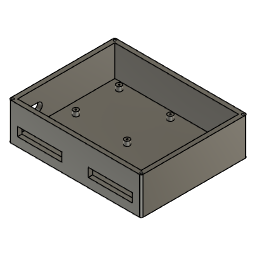
台座 (Autodesk Fusion 360 design; units mm, degrees)
Autodesk Fusion 360 part; units mm, degrees
note: some values were not read from the file. Set by a fixed rule: which sketch regions a step uses.
sketch "スケッチ6" plane through (0, 0, 0) normal (0, 0, 1) x (1, 0, 0)
  line L0 (75, -45) -> (-75, -45)
  line L1 (-75, -45) -> (-75, 75)
  line L2 (-75, 75) -> (75, 75)
  line L3 (75, 75) -> (75, -45)
  line L4 (-200, 0) -> (160, 0)
  dimension "d22" = 150
  dimension "d110" = 75
  dimension "d111" = 45
  constraint horizontal L0
  constraint perpendicular L0 L1
  constraint parallel L0 L2
  constraint parallel L1 L3
  constraint perpendicular L3 L4
  measures "d22" distance of L1.end L2.end
  measures "d110" distance of L2 L4
  measures "d111" distance of L0 L4
extrude "押し出し4" add sketch "スケッチ6" along normal blind 42
sketch "スケッチ7" plane through (0, 0, 42) normal (0, 0, 1) x (-1, 0, 0)
  line L0 (-75, -75) -> (75, -75)
  line L1 (75, -75) -> (75, 45)
  line L2 (75, 45) -> (-75, 45)
  line L3 (-75, 45) -> (-75, -75)
  line L4 (70, -70) -> (-70, -70)
  line L5 (-70, -70) -> (-70, 40)
  line L6 (-70, 40) -> (70, 40)
  line L7 (70, 40) -> (70, -70)
  dimension "d26" = 5
  dimension "d27" = 5
  constraint horizontal L4
  constraint vertical L5
  constraint horizontal L6
  constraint vertical L7
  measures "d26" distance of L2 L6
  measures "d27" distance of L0 L4
extrude "押し出し5" cut sketch "スケッチ7" against normal blind 35 contours L4 L5 L6 L7
sketch "スケッチ8" plane through (0, 0, 7) normal (0, 0, 1) x (-1, 0, 0)
  line L0 (70, 40) -> (-70, 40)
  line L1 (-70, 40) -> (-70, -70)
  line L2 (-70, -70) -> (70, -70)
  line L3 (70, -70) -> (70, 40)
  circle A0 centre (56.5, -61.5) radius 3
  circle A1 centre (-1.5, -61.5) radius 3
  circle A2 centre (56.5, -12.5) radius 3
  circle A3 centre (-1.5, -12.5) radius 3
  dimension "d32" = 6
  dimension "d35" = 6
  dimension "d37" = 58
  dimension "d41" = 6
  dimension "d42" = 6
  measures "d32" diameter of A0
  measures "d35" diameter of A1
  measures "d37" distance of A0.centre A1.centre
  measures "d41" diameter of A2
  measures "d42" diameter of A3
extrude "押し出し6" add sketch "スケッチ8" along normal blind 5 contours A0 | A1 | A2 | A3
sketch "スケッチ9" plane through (0, 0, 12) normal (0, 0, 1) x (-1, 0, 0)
  circle A0 centre (56.5, -61.5) radius 3
  line L0 (56.5, -61.5) -> (53.5, -61.5)
  line L1 (56.5, -61.5) -> (56.5, -64.5)
  constraint coincident A0.centre L0.start
  constraint coincident A0 L0.end
  constraint horizontal L0
  constraint coincident A0 L1.end
  constraint perpendicular L0 L1
hole "穴1" at (-56.5, 61.5, 12) direction (0, 0, -1) diameter 1.623 depth 10 tip angle 118
thread "ねじ1" "ISO Metric profile 2.0 M2x0.4 6H"
sketch "スケッチ10" plane through (0, 0, 12) normal (0, 0, 1) x (-1, 0, 0)
  circle A0 centre (-1.5, -61.5) radius 3
  line L0 (-1.5, -61.5) -> (-3.2909, -61.5)
  line L1 (-3.2909, -61.5) -> (-1.5, -61.5)
  line L2 (-1.5, -61.5) -> (-1.5, -64)
  constraint coincident A0.centre L0.start
  constraint horizontal L0
  constraint perpendicular L0 L2
hole "穴2" at (1.5, 61.5, 12) direction (0, 0, -1) diameter 1.623 depth 10 tip angle 118
thread "ねじ2" "ISO Metric profile 2.0 M2x0.4 6H"
sketch "スケッチ11" plane through (0, 0, 12) normal (0, 0, 1) x (-1, 0, 0)
  circle A0 centre (-1.5, -12.5) radius 3
  line L0 (-1.5, -12.5) -> (-4.5, -12.5)
  line L1 (-1.5, -12.5) -> (-1.5, -15.5)
  constraint coincident A0.centre L0.start
  constraint coincident A0 L0.end
  constraint horizontal L0
  constraint coincident A0 L1.end
  constraint perpendicular L0 L1
hole "穴3" at (1.5, 12.5, 12) direction (0, 0, -1) diameter 1.623 depth 10 tip angle 118
thread "ねじ3" "ISO Metric profile 2.0 M2x0.4 6H"
sketch "スケッチ12" plane through (0, 0, 12) normal (0, 0, 1) x (-1, 0, 0)
  circle A0 centre (56.5, -12.5) radius 3
  line L0 (56.5, -12.5) -> (53.5, -12.5)
  line L1 (56.5, -12.5) -> (56.5, -15.5)
  constraint coincident A0.centre L0.start
  constraint coincident A0 L0.end
  constraint horizontal L0
  constraint coincident A0 L1.end
  constraint perpendicular L0 L1
hole "穴4" at (-56.5, 12.5, 12) direction (0, 0, -1) diameter 1.623 depth 10 tip angle 118
thread "ねじ4" "ISO Metric profile 2.0 M2x0.4 6H"
sketch "スケッチ13" plane through (-75, 0, 0) normal (-1, 0, 0) x (0, -1, 0)
  line L0 (-75, 0) -> (45, 0)
  line L1 (45, 0) -> (45, 42)
  line L2 (45, 42) -> (-75, 42)
  line L3 (-75, 42) -> (-75, 0)
  line L4 (17, 27) -> (32, 27)
  line L5 (32, 17) -> (25.3423, 17)
  arc A0 (32, 17) -> (32, 27) centre (32, 22) ccw
  line L6 (25.3423, 17) -> (17, 17)
  arc A1 (17, 27) -> (17, 17) centre (17, 22) ccw
  dimension "d55" = 15
  dimension "d56" = 10
  constraint horizontal L4
  constraint horizontal L5
  constraint tangent L4 A0
  constraint parallel L5 L6
  constraint tangent L4 A1
  measures "d55" distance of L4.start L4.end
  measures "d56" distance of L4 L5
extrude "押し出し7" cut sketch "スケッチ13" against normal blind 10 contours L4 L5 A0 L6 A1
sketch "スケッチ15" plane through (0, -45, 0) normal (0, -1, 0) x (1, 0, 0)
  line L0 (-75, 0) -> (75, 0)
  line L1 (75, 0) -> (75, 42)
  line L2 (75, 42) -> (-75, 42)
  line L3 (-75, 42) -> (-75, 0)
  line L4 (-15, 10) -> (-65, 10)
  line L5 (-65, 10) -> (-65, 20)
  line L6 (-65, 20) -> (-15, 20)
  line L7 (-15, 20) -> (-15, 10)
  line L8 (15, 20) -> (65, 20)
  line L9 (65, 20) -> (65, 10)
  line L10 (65, 10) -> (15, 10)
  line L11 (15, 10) -> (15, 20)
  constraint horizontal L4
  constraint vertical L5
  constraint horizontal L6
  constraint vertical L7
  constraint horizontal L8
  constraint vertical L9
  constraint horizontal L10
  constraint vertical L11
extrude "押し出し8" cut sketch "スケッチ15" against normal blind 5 contours L4 L5 L6 L7 | L8 L9 L10 L11
sketch "スケッチ16" plane through (0, 0, 42) normal (0, 0, 1) x (-1, 0, 0)
  line L0 (-70, -70) -> (-70, 40)
  line L1 (-70, 40) -> (70, 40)
  line L2 (70, 40) -> (70, -70)
  line L3 (70, -70) -> (-70, -70)
  line L4 (-75, -75) -> (75, -75)
  line L5 (75, -75) -> (75, 45)
  line L6 (75, 45) -> (-75, 45)
  line L7 (-75, 45) -> (-75, -75)
  circle A0 centre (72.5, -72.5) radius 1.5
  circle A1 centre (-72.5, -72.5) radius 1.5
  circle A2 centre (72.5, 72.5) radius 1.5
  circle A3 centre (-72.5, 72.5) radius 1.5
  dimension "d96" = 3
  dimension "d97" = 2.5
  dimension "d98" = 2.5
  measures "d96" diameter of A0
  measures "d97" distance of L4 A0.centre
  measures "d98" distance of L5 A0.centre
hole "穴5" at (-72.5, 72.5, 42) at (-72.5, -72.5, 42) at (72.5, 72.5, 42) at (72.5, -72.5, 42) direction (0, 0, -1) diameter 2.529 depth 10 tip angle 118
thread "ねじ5" "ISO Metric profile 3.0 M3x0.5 6H"
sketch "スケッチ17" plane through (0, 0, 0) normal (0, 0, 1) x (1, 0, 0)
  circle A0 centre (0, 45) radius 11.95
  circle A1 centre (0, -15) radius 11.95
  line L0 (-75, 75) -> (75, 75)
  line L1 (75, -45) -> (-75, -45)
  dimension "d102" = 23.9
  dimension "d103" = 23.9
  dimension "d104" = 30
  dimension "d105" = 30
  measures "d102" diameter of A0
  measures "d103" diameter of A1
  measures "d104" distance of A0.centre L0
  measures "d105" distance of A1.centre L1
extrude "押し出し9" cut sketch "スケッチ17" along normal blind 5
fillet "フィレット1" radius 2 4 edges at (75, -45, 21) (-75, -45, 21) (75, 75, 21) (-75, 75, 21)
sketch "スケッチ18" plane through (0, 0, 42) normal (0, 0, 1) x (-1, 0, 0)
  arc A0 (73, -75) -> (75, -73) centre (73, -73) ccw
  line L0 (75, -73) -> (75, 43)
  arc A1 (75, 43) -> (73, 45) centre (73, 43) ccw
  line L1 (73, 45) -> (-73, 45)
  arc A2 (-73, 45) -> (-75, 43) centre (-73, 43) ccw
  line L2 (-75, 43) -> (-75, -73)
  arc A3 (-75, -73) -> (-73, -75) centre (-73, -73) ccw
  line L3 (-73, -75) -> (73, -75)
  circle A4 centre (-72.5, -72.5) radius 1.2645
  circle A5 centre (72.5, -72.5) radius 1.2645
  line L4 (-70, -70) -> (-70, 40)
  line L5 (-70, 40) -> (70, 40)
  line L6 (70, 40) -> (70, -70)
  line L7 (70, -70) -> (-70, -70)
  circle A6 centre (72.5, 42.5) radius 1
  circle A7 centre (-72.5, 42.5) radius 1
  dimension "d112" = 2
  dimension "d113" = 2.5
  dimension "d114" = 2.5
  dimension "d115" = 2
  dimension "d116" = 2.5
  dimension "d117" = 2.5
  measures "d112" diameter of A6
  measures "d113" distance of L1 A6.centre
  measures "d114" distance of L0 A6.centre
  measures "d115" diameter of A7
  measures "d116" distance of L2 A7.centre
  measures "d117" distance of L1 A7.centre
hole "穴6" at (-72.5, -42.5, 42) at (72.5, -42.5, 42) direction (0, 0, -1) diameter 2.529 depth 10 tip angle 118
thread "ねじ6" "ISO Metric profile 3.0 M3x0.5 6H"
equation "d111 = 75 mm - 30 mm"
